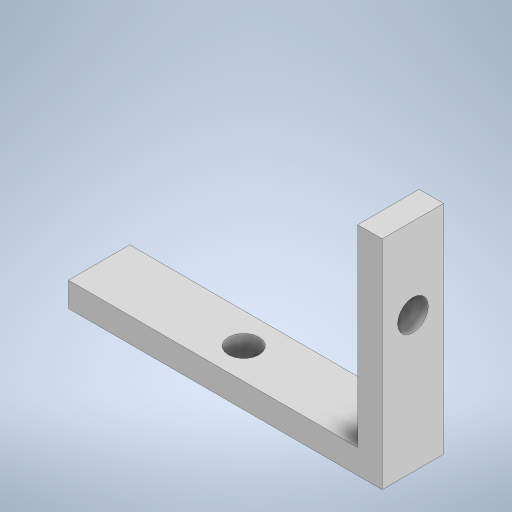
# Autodesk Inventor part: 베벨기어 003
Saved by Autodesk Inventor 2023 (Build 270158000, 158)
## iProperties
Created: 2022-06-18
Part Number: 베벨기어 003
Material: 일반
Document SubType Name: Modeling
Designer: fly01
Density: 1 g/cm^3
Appearance: 기본값
Author: fly01
Autodesk Inventor part; units mm, degrees
ref_plane "YZ Plane" through (0, 0, 0) normal (1, 0, 0) x (0, 1, 0)
ref_plane "XZ Plane" through (0, 0, 0) normal (0, 1, 0) x (-1, 0, 0)
ref_plane "XY Plane" through (0, 0, 0) normal (0, 0, 1) x (1, 0, 0)
sketch "스케치1" plane through (0, 0, 0) normal (0, 0, 1) x (1, 0, 0)
  line L0 (0, 0) -> (47.183, 0)
  line L1 (47.183, 0) -> (47.183, -4)
  line L2 (47.183, -4) -> (0, -4)
  line L3 (0, -4) -> (0, 0)
  line L4 (47.183, -4) -> (51.183, -4)
  line L5 (51.183, -4) -> (51.183, 31.431)
  line L6 (51.183, 31.431) -> (47.183, 31.431)
  line L7 (47.183, 31.431) -> (47.183, -4)
  point P0 (47.183, 0)
  dimension "d0" = 47.183
  dimension "d1" = 31.431
  dimension "d2" = 4
  dimension "d3" = 4
  constraints: 16 end point, 4 parallel, 2 horizontal, 2 perpendicular
  measures "d0" distance of L0.start L0.end
  measures "d1" distance between parallel lines of L6 L0
  measures "d2" distance of L5.end L6.end
  measures "d3" distance of L2.end L0.start
extrude "돌출1" add sketch "스케치1" along normal blind 10
sketch "스케치2" plane through (0, 0, 0) normal (0, 1, 0) x (1, 0, 0)
  line L0 (0, 0) -> (0, -10) projected
  line L1 (0, -5) -> (47.183, -5) construction
  line L2 (47.183, 0) -> (47.183, -10) projected
  circle A0 centre (23.5915, -5) radius 2.5
  dimension "d6" = 5
  constraints: 3 midpoint, 2 end point, 1 centre point
  measures "d6" diameter of A0
extrude "돌출2" cut sketch "스케치2" against normal blind 9.25
sketch "스케치3" plane through (47.183, 0, 0) normal (-1, 0, 0) x (0, 0, 1)
  line L0 (0, 31.431) -> (10, 31.431) projected
  line L1 (5, 31.431) -> (5, 4.931)
  circle A0 centre (5, 18.181) radius 2.5
  point P0 (0, 0)
  dimension "d9" = 5
  constraints: 2 end point, 2 midpoint, 1 centre point, 1 vertical
  measures "d9" diameter of A0
extrude "돌출3" cut sketch "스케치3" against normal blind 8.75
